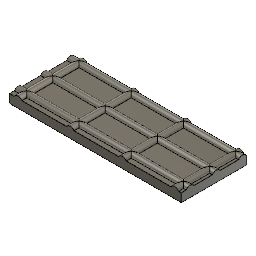
Door2 v2 (Autodesk Fusion 360 design; units mm, degrees)
Autodesk Fusion 360 part; units mm, degrees
box "BoxPrimitive1" add length 15 width 39.5 height 2 placed x (0, 0, 1) y (1, 0, 0) z (0, 1, 0) at (0, 0, 0)
sketch "Sketch2" plane through (0, 0, 0) normal (1, 0, 0) x (0, 0, -1)
cylinder "CylinderPrimitive1" add diameter 2 height 39.5 placed x (0, 0, -1) y (0, 1, 0) z (1, 0, 0) at (0, 1.5, 1)
cylinder "CylinderPrimitive2" add diameter 2 height -39.5 placed x (0, 0, -1) y (0, 1, 0) z (1, 0, 0) at (39.5, 1.5, 7)
cylinder "CylinderPrimitive3" add diameter 2 height -39.5 placed x (0, 0, -1) y (0, 1, 0) z (1, 0, 0) at (39.5, 1.5, 13)
cylinder "CylinderPrimitive4" add diameter 2 height -15 placed x (0, 1, 0) y (1, 0, 0) z (0, 0, -1) at (2, 1.5, 0)
cylinder "CylinderPrimitive6" add diameter 2 height -15 placed x (0, 1, 0) y (1, 0, 0) z (0, 0, -1) at (14, 1.5, 0)
cylinder "CylinderPrimitive8" add diameter 2 height -15 placed x (0, 1, 0) y (1, 0, 0) z (0, 0, -1) at (26, 1.5, 0)
cylinder "CylinderPrimitive10" add diameter 2 height -15 placed x (0, 1, 0) y (1, 0, 0) z (0, 0, -1) at (38, 1.5, 0)
